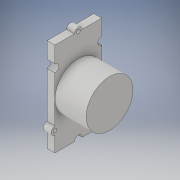
# Autodesk Inventor part: Grove - Oxygen Sensor
Saved by Autodesk Inventor 2018 (Build 220112000, 112)
## iProperties
Created: 2018-01-27
Part Number: Grove - Oxygen Sensor
Material: Všeobecné
Document SubType Name: Modeling
Designer: Kuba
Density: 1 g/cm^3
Appearance: Výchozí
Author: Kuba
Autodesk Inventor part; units mm, degrees
ref_plane "YZ Plane" through (0, 0, 0) normal (1, 0, 0) x (0, 1, 0)
ref_plane "XZ Plane" through (0, 0, 0) normal (0, 1, 0) x (-1, 0, 0)
ref_plane "XY Plane" through (0, 0, 0) normal (0, 0, 1) x (1, 0, 0)
sketch "Náčrt1" plane through (0, 0, 0) normal (1, 0, 0) x (0, 1, 0)
  arc A0 (12, -4) -> (12, -6) centre (12, -5) ccw
  arc A1 (0, -6.1587) -> (0, -4.1587) centre (0, -5.1587) ccw
  arc A2 (12, -20) -> (12, -18) centre (12, -19) ccw
  arc A3 (0, -18) -> (0, -20) centre (0, -19) ccw
  line L0 (0, -4.1587) -> (0, 0)
  line L1 (12, 0) -> (12, -4)
  line L2 (12, -6) -> (12, -18)
  line L3 (12, -20) -> (12, -24)
  line L4 (0, -24) -> (0, -20)
  line L5 (0, -18) -> (0, -6.1587)
  circle A4 centre (12, -19) radius 0.5002
  circle A5 centre (0, -19) radius 0.5002
  arc A6 (7, 0) -> (5, 0) centre (6, 0) ccw
  line L6 (0, 0) -> (5, 0)
  line L7 (7, 0) -> (12, 0)
  circle A7 centre (6, 0) radius 0.5
  arc A8 (7, -24) -> (5, -24) centre (6, -24) ccw
  line L8 (12, -24) -> (7, -24)
  line L9 (5, -24) -> (0, -24)
  dimension "d0" = 12
  dimension "d1" = 24
  dimension "d2" = 2
  dimension "d3" = 2
  dimension "d4" = 5
  dimension "d5" = 5
  dimension "d6" = 5
  dimension "d7" = 2
  dimension "d8" = 1
  constraints: 20 end point, 13 parallel, 12 point on circle, 9 centre point, 6 perpendicular, 3 coincident, 2 horizontal
  measures "d0" distance of L0.end L1.start
  measures "d1" distance of L4.start L0.end
  measures "d2" diameter of A0
  measures "d3" diameter of A1
  measures "d4" distance of L1.start A0.centre
  measures "d5" distance of L3.end A2.centre
  measures "d6" distance of L4.start A3.centre
  measures "d7" diameter of A6
  measures "d8" diameter of A7
extrude "Vysunutí1" add sketch "Náčrt1" along normal blind 2
sketch "Náčrt2" plane through (2, 0, 0) normal (1, 0, 0) x (0, 0, -1)
  circle A0 centre (12, 6.016) radius 6
  arc A1 (24, 7) -> (24, 5) centre (24, 6) ccw projected
  point P0 (0, 0)
  dimension "d11" = 12
  dimension "d12" = 12
  constraints: 1 centre point
  measures "d11" diameter of A0
  measures "d12" distance of A1.centre A0.centre
extrude "Vysunutí2" add sketch "Náčrt2" along normal blind 8
equation "\"d6\" = d5"
